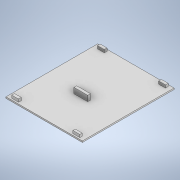
# Autodesk Inventor part: bottomplate
Saved by Autodesk Inventor 2021 (Build 250183000, 183)
## iProperties
Created: 2021-05-05
Part Number: bottomplate
Material: Generic
Document SubType Name: Modeling
Designer: email
Density: 1 g/cm^3
Appearance: Default
Author: email
Autodesk Inventor part; units mm, degrees
ref_plane "YZ Plane" through (0, 0, 0) normal (1, 0, 0) x (0, 1, 0)
ref_plane "XZ Plane" through (0, 0, 0) normal (0, 1, 0) x (-1, 0, 0)
ref_plane "XY Plane" through (0, 0, 0) normal (0, 0, 1) x (1, 0, 0)
sketch "Sketch1" plane through (0, 0, 0) normal (0, 1, 0) x (-1, 0, 0)
  line L0 (27.775, -33.32) -> (-27.775, -33.32)
  line L1 (-27.775, -33.32) -> (-27.775, 33.32)
  line L2 (-27.775, 33.32) -> (27.775, 33.32)
  line L3 (27.775, 33.32) -> (27.775, -33.32)
  line L4 (27.775, -33.32) -> (-27.775, 33.32) construction
  line L5 (-27.775, -33.32) -> (27.775, 33.32) construction
  line L6 (26.775, -32.3) -> (-26.775, -32.3)
  line L7 (-26.775, -32.3) -> (-26.775, 32.3)
  line L8 (-26.775, 32.3) -> (26.775, 32.3)
  line L9 (26.775, 32.3) -> (26.775, -32.3)
  line L10 (26.775, -32.3) -> (-26.775, 32.3) construction
  line L11 (-26.775, -32.3) -> (26.775, 32.3) construction
  point P0 (0, 0)
  dimension "d0" = 66.64
  dimension "d1" = 55.55
  dimension "d2" = 64.6
  dimension "d3" = 53.55
  constraints: 24 end point, 4 midpoint, 4 parallel, 2 horizontal, 2 perpendicular
  measures "d0" distance of L0.end L1.end
  measures "d1" distance of L1.end L2.end
  measures "d2" distance of L6.end L7.end
  measures "d3" distance of L6.start L6.end
extrude "Extrusion1" add sketch "Sketch1" along normal blind 1 contours L0 L1 L2 L3 | L6 L7 L8 L9
sketch "Sketch2" plane through (0, 1, 0) normal (0, 1, 0) x (1, 0, 0)
  line L0 (-26.775, 32.15) -> (26.775, 32.15)
  line L1 (26.775, 32.15) -> (26.775, -32.15)
  line L2 (26.775, -32.15) -> (-26.775, -32.15)
  line L3 (-26.775, -32.15) -> (-26.775, 32.15)
  line L4 (-26.775, 32.15) -> (26.775, -32.15) construction
  line L5 (26.775, 32.15) -> (-26.775, -32.15) construction
  line L6 (-26.775, 32.15) -> (-24.775, 32.15)
  line L7 (-24.775, 32.15) -> (-24.775, 30.15)
  line L8 (-24.775, 30.15) -> (-26.775, 30.15) construction
  line L9 (-26.775, 30.15) -> (-26.775, 32.15)
  line L10 (-24.775, 30.15) -> (-19.775, 30.15)
  line L11 (-19.775, 30.15) -> (-19.775, 32.15)
  line L12 (-19.775, 32.15) -> (-24.775, 32.15)
  line L13 (-24.775, 32.15) -> (-24.775, 30.15)
  line L14 (26.775, 32.15) -> (24.775, 32.15)
  line L15 (24.775, 32.15) -> (24.775, 30.15)
  line L16 (24.775, 30.15) -> (26.775, 30.15) construction
  line L17 (26.775, 30.15) -> (26.775, 32.15)
  line L18 (24.775, 32.15) -> (19.775, 32.15)
  line L19 (19.775, 32.15) -> (19.775, 30.15)
  line L20 (19.775, 30.15) -> (24.775, 30.15)
  line L21 (24.775, 30.15) -> (24.775, 32.15)
  line L22 (-26.775, -32.15) -> (-24.775, -32.15)
  line L23 (-24.775, -32.15) -> (-24.775, -30.15)
  line L24 (-24.775, -30.15) -> (-26.775, -30.15) construction
  line L25 (-26.775, -30.15) -> (-26.775, -32.15)
  line L26 (-24.775, -30.15) -> (-19.775, -30.15)
  line L27 (-19.775, -30.15) -> (-19.775, -32.15)
  line L28 (-19.775, -32.15) -> (-24.775, -32.15)
  line L29 (-24.775, -32.15) -> (-24.775, -30.15)
  line L30 (26.775, -32.15) -> (24.775, -32.15)
  line L31 (24.775, -32.15) -> (24.775, -30.45)
  line L32 (24.775, -30.45) -> (26.775, -30.45) construction
  line L33 (26.775, -30.45) -> (26.775, -32.15)
  line L34 (24.775, -30.45) -> (19.775, -30.45)
  line L35 (19.775, -30.45) -> (19.775, -32.15)
  line L36 (19.775, -32.15) -> (24.775, -32.15)
  line L37 (24.775, -32.15) -> (24.775, -30.45)
  point P0 (0, 0)
  point P1 (-24.775, -32.15)
  point P2 (-24.775, 32.15)
  dimension "d6" = 53.55
  dimension "d7" = 64.3
  dimension "d8" = 2
  dimension "d9" = 2
  dimension "d10" = 5
  dimension "d11" = 2
  dimension "d12" = 2
  dimension "d13" = 5
  dimension "d14" = 2
  dimension "d15" = 2
  dimension "d16" = 5
  dimension "d17" = 2
  dimension "d18" = 5
  constraints: 76 end point, 18 parallel, 9 horizontal, 9 perpendicular, 3 point on line, 2 midpoint
  measures "d6" distance of L0.start L0.end
  measures "d7" distance of L0.end L1.end
  measures "d8" distance of L6.end L7.end
  measures "d9" distance of L7.end L8.end
  measures "d10" distance of L7.end L10.end
  measures "d11" distance of L15.end L16.end
  measures "d12" distance of L14.end L15.end
  measures "d13" distance of L19.end L20.end
  measures "d14" distance of L22.end L23.end
  measures "d15" distance of L23.end L24.end
  measures "d16" distance of L23.end L26.end
  measures "d17" distance of L31.end L32.end
  measures "d18" distance of L31.end L34.end
extrude "Extrusion2" add sketch "Sketch2" along normal blind 2 contours L0 L11 L10 L7 | L0 L15 L20 L19 | L23 L26 L27 L2 | L35 L34 L31 L2
sketch "Sketch3" plane through (0, 1, 0) normal (0, 1, 0) x (1, 0, 0)
  line L0 (27.775, 33.32) -> (-27.775, 33.32) projected
  line L1 (0, 33.32) -> (0, -4.68)
  line L2 (0, -4.68) -> (5, -4.68)
  line L3 (0, -4.68) -> (-5, -4.68)
  line L4 (-5, -4.68) -> (-5, -6.68)
  line L5 (-5, -6.68) -> (5, -6.68)
  line L6 (5, -6.68) -> (5, -4.68)
  point P0 (0, 0)
  dimension "d21" = 38
  dimension "d22" = 5
  dimension "d23" = 5
  dimension "d24" = 2
  constraints: 12 end point, 3 horizontal, 2 vertical, 1 midpoint, 1 perpendicular
  measures "d21" distance of L1.start L1.end
  measures "d22" distance of L1.end L3.end
  measures "d23" distance of L1.end L2.end
  measures "d24" distance of L3.end L4.end
extrude "Extrusion3" add sketch "Sketch3" along normal blind 4
body "Solid1"
